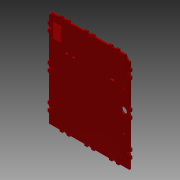
# Autodesk Inventor part: dolna_gt2_v2ipt
Saved by Autodesk Inventor 2013 (Build 170138000, 138)
## iProperties
Created: 2014-01-08
Part Number: dolna_gt2_v2ipt
Material: Generic
Document SubType Name: Modeling
Designer: dzban
Density: 1 g/cm^3
Author: dzban
Autodesk Inventor part; units mm, degrees
ref_plane "YZ Plane" through (0, 0, 0) normal (1, 0, 0) x (0, 1, 0)
ref_plane "XZ Plane" through (0, 0, 0) normal (0, 1, 0) x (-1, 0, 0)
ref_plane "XY Plane" through (0, 0, 0) normal (0, 0, 1) x (1, 0, 0)
sketch "Sketch1" plane through (0, 0, 0) normal (0, 1, 0) x (-1, 0, 0)
  line L0 (324.1317, 450.5892) -> (324.1317, 456.9892)
  line L1 (324.1317, 456.9892) -> (336.1317, 456.9892)
  line L2 (336.1317, 456.9892) -> (336.1317, 450.5892)
  line L3 (336.1317, 450.5892) -> (324.1317, 450.5892)
  line L4 (351.7317, 450.5892) -> (351.7317, 456.9892)
  line L5 (351.7317, 456.9892) -> (363.7317, 456.9892)
  line L6 (363.7317, 456.9892) -> (363.7317, 450.5892)
  line L7 (363.7317, 450.5892) -> (351.7317, 450.5892)
  arc A0 (416.5867, 566.9892) -> (427.5867, 555.9892) centre (427.5867, 566.9892) ccw
  line L8 (416.5867, 566.9892) -> (384.9367, 566.9892)
  line L9 (384.9367, 566.9892) -> (384.6367, 572.9892)
  line L10 (384.6367, 572.9892) -> (372.8367, 572.9892)
  line L11 (372.8367, 572.9892) -> (372.5367, 566.9892)
  line L12 (372.5367, 566.9892) -> (366.4367, 566.9892)
  line L13 (366.4367, 566.9892) -> (366.4367, 559.9892)
  line L14 (366.4367, 559.9892) -> (367.6867, 559.9892)
  line L15 (367.6867, 559.9892) -> (367.6867, 558.1892)
  line L16 (367.6867, 558.1892) -> (366.4367, 558.1892)
  line L17 (366.4367, 558.1892) -> (366.4367, 556.3892)
  line L18 (366.4367, 556.3892) -> (363.4367, 556.3892)
  line L19 (363.4367, 556.3892) -> (363.4367, 558.1892)
  line L20 (363.4367, 558.1892) -> (362.1867, 558.1892)
  line L21 (362.1867, 558.1892) -> (362.1867, 559.9892)
  line L22 (362.1867, 559.9892) -> (363.4367, 559.9892)
  line L23 (363.4367, 559.9892) -> (363.4367, 566.9892)
  line L24 (363.4367, 566.9892) -> (357.3367, 566.9892)
  line L25 (357.3367, 566.9892) -> (357.0367, 572.9892)
  line L26 (357.0367, 572.9892) -> (345.2367, 572.9892)
  line L27 (345.2367, 572.9892) -> (344.9367, 566.9892)
  line L28 (344.9367, 566.9892) -> (284.9367, 566.9892)
  line L29 (284.9367, 566.9892) -> (284.6367, 572.9892)
  line L30 (284.6367, 572.9892) -> (272.8367, 572.9892)
  line L31 (272.8367, 572.9892) -> (272.5367, 566.9892)
  line L32 (272.5367, 566.9892) -> (266.4367, 566.9892)
  line L33 (266.4367, 566.9892) -> (266.4367, 559.9892)
  line L34 (266.4367, 559.9892) -> (267.6867, 559.9892)
  line L35 (267.6867, 559.9892) -> (267.6867, 558.1892)
  line L36 (267.6867, 558.1892) -> (266.4367, 558.1892)
  line L37 (266.4367, 558.1892) -> (266.4367, 556.3892)
  line L38 (266.4367, 556.3892) -> (263.4367, 556.3892)
  line L39 (263.4367, 556.3892) -> (263.4367, 558.1892)
  line L40 (263.4367, 558.1892) -> (262.1867, 558.1892)
  line L41 (262.1867, 558.1892) -> (262.1867, 559.9892)
  line L42 (262.1867, 559.9892) -> (263.4367, 559.9892)
  line L43 (263.4367, 559.9892) -> (263.4367, 566.9892)
  line L44 (263.4367, 566.9892) -> (257.3367, 566.9892)
  line L45 (257.3367, 566.9892) -> (257.0367, 572.9892)
  line L46 (257.0367, 572.9892) -> (245.2367, 572.9892)
  line L47 (245.2367, 572.9892) -> (244.9367, 566.9892)
  line L48 (244.9367, 566.9892) -> (184.9367, 566.9892)
  line L49 (184.9367, 566.9892) -> (184.6367, 572.9892)
  line L50 (184.6367, 572.9892) -> (172.8367, 572.9892)
  line L51 (172.8367, 572.9892) -> (172.5367, 566.9892)
  line L52 (172.5367, 566.9892) -> (166.4367, 566.9892)
  line L53 (166.4367, 566.9892) -> (166.4367, 559.9892)
  line L54 (166.4367, 559.9892) -> (167.6867, 559.9892)
  line L55 (167.6867, 559.9892) -> (167.6867, 558.1892)
  line L56 (167.6867, 558.1892) -> (166.4367, 558.1892)
  line L57 (166.4367, 558.1892) -> (166.4367, 556.3892)
  line L58 (166.4367, 556.3892) -> (163.4367, 556.3892)
  line L59 (163.4367, 556.3892) -> (163.4367, 558.1892)
  line L60 (163.4367, 558.1892) -> (162.1867, 558.1892)
  line L61 (162.1867, 558.1892) -> (162.1867, 559.9892)
  line L62 (162.1867, 559.9892) -> (163.4367, 559.9892)
  line L63 (163.4367, 559.9892) -> (163.4367, 566.9892)
  line L64 (163.4367, 566.9892) -> (157.3367, 566.9892)
  line L65 (157.3367, 566.9892) -> (157.0367, 572.9892)
  line L66 (157.0367, 572.9892) -> (145.2367, 572.9892)
  line L67 (145.2367, 572.9892) -> (144.9367, 566.9892)
  line L68 (144.9367, 566.9892) -> (118.2867, 566.9892)
  arc A1 (102.2867, 550.9892) -> (118.2867, 566.9892) centre (102.2867, 566.9892) ccw
  line L69 (102.2867, 550.9892) -> (102.2867, 529.3892)
  line L70 (102.2867, 529.3892) -> (96.2867, 529.0892)
  line L71 (96.2867, 529.0892) -> (96.2867, 517.2892)
  line L72 (96.2867, 517.2892) -> (102.2867, 516.9892)
  line L73 (102.2867, 516.9892) -> (102.2867, 510.8892)
  line L74 (102.2867, 510.8892) -> (109.2867, 510.8892)
  line L75 (109.2867, 510.8892) -> (109.2867, 512.1392)
  line L76 (109.2867, 512.1392) -> (111.0867, 512.1392)
  line L77 (111.0867, 512.1392) -> (111.0867, 510.8892)
  line L78 (111.0867, 510.8892) -> (112.8867, 510.8892)
  line L79 (112.8867, 510.8892) -> (112.8867, 507.8892)
  line L80 (112.8867, 507.8892) -> (111.0867, 507.8892)
  line L81 (111.0867, 507.8892) -> (111.0867, 506.6392)
  line L82 (111.0867, 506.6392) -> (109.2867, 506.6392)
  line L83 (109.2867, 506.6392) -> (109.2867, 507.8892)
  line L84 (109.2867, 507.8892) -> (102.2867, 507.8892)
  line L85 (102.2867, 507.8892) -> (102.2867, 501.7892)
  line L86 (102.2867, 501.7892) -> (96.2867, 501.4892)
  line L87 (96.2867, 501.4892) -> (96.2867, 489.6892)
  line L88 (96.2867, 489.6892) -> (102.2867, 489.3892)
  line L89 (102.2867, 489.3892) -> (102.2867, 389.3892)
  line L90 (102.2867, 389.3892) -> (96.2867, 389.0892)
  line L91 (96.2867, 389.0892) -> (96.2867, 377.2892)
  line L92 (96.2867, 377.2892) -> (102.2867, 376.9892)
  line L93 (102.2867, 376.9892) -> (102.2867, 370.8892)
  line L94 (102.2867, 370.8892) -> (105.2867, 370.8892)
  line L95 (105.2867, 370.8892) -> (105.2867, 372.1392)
  line L96 (105.2867, 372.1392) -> (107.1867, 372.1392)
  line L97 (107.1867, 372.1392) -> (107.1867, 370.8892)
  line L98 (107.1867, 370.8892) -> (108.8867, 370.8892)
  line L99 (108.8867, 370.8892) -> (108.8867, 367.8892)
  line L100 (108.8867, 367.8892) -> (107.1867, 367.8892)
  line L101 (107.1867, 367.8892) -> (107.1867, 366.6392)
  line L102 (107.1867, 366.6392) -> (105.2867, 366.6392)
  line L103 (105.2867, 366.6392) -> (105.2867, 367.8892)
  line L104 (105.2867, 367.8892) -> (102.2867, 367.8892)
  line L105 (102.2867, 367.8892) -> (102.2867, 361.7892)
  line L106 (102.2867, 361.7892) -> (96.2867, 361.4892)
  line L107 (96.2867, 361.4892) -> (96.2867, 349.6892)
  line L108 (96.2867, 349.6892) -> (102.2867, 349.3892)
  line L109 (102.2867, 349.3892) -> (102.2867, 249.3892)
  line L110 (102.2867, 249.3892) -> (96.2867, 249.0892)
  line L111 (96.2867, 249.0892) -> (96.2867, 237.2892)
  line L112 (96.2867, 237.2892) -> (102.2867, 236.9892)
  line L113 (102.2867, 236.9892) -> (102.2867, 230.8892)
  line L114 (102.2867, 230.8892) -> (109.2867, 230.8892)
  line L115 (109.2867, 230.8892) -> (109.2867, 232.1392)
  line L116 (109.2867, 232.1392) -> (111.0867, 232.1392)
  line L117 (111.0867, 232.1392) -> (111.0867, 230.8892)
  line L118 (111.0867, 230.8892) -> (112.8867, 230.8892)
  line L119 (112.8867, 230.8892) -> (112.8867, 227.8892)
  line L120 (112.8867, 227.8892) -> (111.0867, 227.8892)
  line L121 (111.0867, 227.8892) -> (111.0867, 226.6392)
  line L122 (111.0867, 226.6392) -> (109.2867, 226.6392)
  line L123 (109.2867, 226.6392) -> (109.2867, 227.8892)
  line L124 (109.2867, 227.8892) -> (102.2867, 227.8892)
  line L125 (102.2867, 227.8892) -> (102.2867, 221.7892)
  line L126 (102.2867, 221.7892) -> (96.2867, 221.4892)
  line L127 (96.2867, 221.4892) -> (96.2867, 209.6892)
  line L128 (96.2867, 209.6892) -> (102.2867, 209.3892)
  line L129 (102.2867, 209.3892) -> (102.2867, 171.7892)
  line L130 (102.2867, 171.7892) -> (144.9367, 171.7892)
  line L131 (144.9367, 171.7892) -> (145.2367, 165.7892)
  line L132 (145.2367, 165.7892) -> (157.0367, 165.7892)
  line L133 (157.0367, 165.7892) -> (157.3367, 171.7892)
  line L134 (157.3367, 171.7892) -> (163.4367, 171.7892)
  line L135 (163.4367, 171.7892) -> (163.4367, 178.7892)
  line L136 (163.4367, 178.7892) -> (162.1867, 178.7892)
  line L137 (162.1867, 178.7892) -> (162.1867, 180.5892)
  line L138 (162.1867, 180.5892) -> (163.4367, 180.5892)
  line L139 (163.4367, 180.5892) -> (163.4367, 182.3892)
  line L140 (163.4367, 182.3892) -> (166.4367, 182.3892)
  line L141 (166.4367, 182.3892) -> (166.4367, 180.5892)
  line L142 (166.4367, 180.5892) -> (167.6867, 180.5892)
  line L143 (167.6867, 180.5892) -> (167.6867, 178.7892)
  line L144 (167.6867, 178.7892) -> (166.4367, 178.7892)
  line L145 (166.4367, 178.7892) -> (166.4367, 171.7892)
  line L146 (166.4367, 171.7892) -> (172.5367, 171.7892)
  line L147 (172.5367, 171.7892) -> (172.8367, 165.7892)
  line L148 (172.8367, 165.7892) -> (184.6367, 165.7892)
  line L149 (184.6367, 165.7892) -> (184.9367, 171.7892)
  line L150 (184.9367, 171.7892) -> (244.9367, 171.7892)
  line L151 (244.9367, 171.7892) -> (245.2367, 165.7892)
  line L152 (245.2367, 165.7892) -> (257.0367, 165.7892)
  line L153 (257.0367, 165.7892) -> (257.3367, 171.7892)
  line L154 (257.3367, 171.7892) -> (263.4367, 171.7892)
  line L155 (263.4367, 171.7892) -> (263.4367, 178.7892)
  line L156 (263.4367, 178.7892) -> (262.1867, 178.7892)
  line L157 (262.1867, 178.7892) -> (262.1867, 180.5892)
  line L158 (262.1867, 180.5892) -> (263.4367, 180.5892)
  line L159 (263.4367, 180.5892) -> (263.4367, 182.3892)
  line L160 (263.4367, 182.3892) -> (266.4367, 182.3892)
  line L161 (266.4367, 182.3892) -> (266.4367, 180.5892)
  line L162 (266.4367, 180.5892) -> (267.6867, 180.5892)
  line L163 (267.6867, 180.5892) -> (267.6867, 178.7892)
  line L164 (267.6867, 178.7892) -> (266.4367, 178.7892)
  line L165 (266.4367, 178.7892) -> (266.4367, 171.7892)
  line L166 (266.4367, 171.7892) -> (272.5367, 171.7892)
  line L167 (272.5367, 171.7892) -> (272.8367, 165.7892)
  line L168 (272.8367, 165.7892) -> (284.6367, 165.7892)
  line L169 (284.6367, 165.7892) -> (284.9367, 171.7892)
  line L170 (284.9367, 171.7892) -> (344.9367, 171.7892)
  line L171 (344.9367, 171.7892) -> (345.2367, 165.7892)
  line L172 (345.2367, 165.7892) -> (357.0367, 165.7892)
  line L173 (357.0367, 165.7892) -> (357.3367, 171.7892)
  line L174 (357.3367, 171.7892) -> (363.4367, 171.7892)
  line L175 (363.4367, 171.7892) -> (363.4367, 178.7892)
  line L176 (363.4367, 178.7892) -> (362.1867, 178.7892)
  line L177 (362.1867, 178.7892) -> (362.1867, 180.5892)
  line L178 (362.1867, 180.5892) -> (363.4367, 180.5892)
  line L179 (363.4367, 180.5892) -> (363.4367, 182.3892)
  line L180 (363.4367, 182.3892) -> (366.4367, 182.3892)
  line L181 (366.4367, 182.3892) -> (366.4367, 180.5892)
  line L182 (366.4367, 180.5892) -> (367.6867, 180.5892)
  line L183 (367.6867, 180.5892) -> (367.6867, 178.7892)
  line L184 (367.6867, 178.7892) -> (366.4367, 178.7892)
  line L185 (366.4367, 178.7892) -> (366.4367, 171.7892)
  line L186 (366.4367, 171.7892) -> (372.5367, 171.7892)
  line L187 (372.5367, 171.7892) -> (372.8367, 165.7892)
  line L188 (372.8367, 165.7892) -> (384.6367, 165.7892)
  line L189 (384.6367, 165.7892) -> (384.9367, 171.7892)
  line L190 (384.9367, 171.7892) -> (427.5867, 171.7892)
  line L191 (427.5867, 171.7892) -> (427.5867, 209.3892)
  line L192 (427.5867, 209.3892) -> (433.5867, 209.6892)
  line L193 (433.5867, 209.6892) -> (433.5867, 221.4892)
  line L194 (433.5867, 221.4892) -> (427.5867, 221.7892)
  line L195 (427.5867, 221.7892) -> (427.5867, 227.8892)
  line L196 (427.5867, 227.8892) -> (420.5867, 227.8892)
  line L197 (420.5867, 227.8892) -> (420.5867, 226.6392)
  line L198 (420.5867, 226.6392) -> (418.7867, 226.6392)
  line L199 (418.7867, 226.6392) -> (418.7867, 227.8892)
  line L200 (418.7867, 227.8892) -> (416.9867, 227.8892)
  line L201 (416.9867, 227.8892) -> (416.9867, 230.8892)
  line L202 (416.9867, 230.8892) -> (418.7867, 230.8892)
  line L203 (418.7867, 230.8892) -> (418.7867, 232.1392)
  line L204 (418.7867, 232.1392) -> (420.5867, 232.1392)
  line L205 (420.5867, 232.1392) -> (420.5867, 230.8892)
  line L206 (420.5867, 230.8892) -> (427.5867, 230.8892)
  line L207 (427.5867, 230.8892) -> (427.5867, 236.9892)
  line L208 (427.5867, 236.9892) -> (433.5867, 237.2892)
  line L209 (433.5867, 237.2892) -> (433.5867, 249.0892)
  line L210 (433.5867, 249.0892) -> (427.5867, 249.3892)
  line L211 (427.5867, 249.3892) -> (427.5867, 349.3892)
  line L212 (427.5867, 349.3892) -> (433.5867, 349.6892)
  line L213 (433.5867, 349.6892) -> (433.5867, 361.4892)
  line L214 (433.5867, 361.4892) -> (427.5867, 361.7892)
  line L215 (427.5867, 361.7892) -> (427.5867, 367.8892)
  line L216 (427.5867, 367.8892) -> (420.5867, 367.8892)
  line L217 (420.5867, 367.8892) -> (420.5867, 366.6392)
  line L218 (420.5867, 366.6392) -> (418.7867, 366.6392)
  line L219 (418.7867, 366.6392) -> (418.7867, 367.8892)
  line L220 (418.7867, 367.8892) -> (416.9867, 367.8892)
  line L221 (416.9867, 367.8892) -> (416.9867, 370.8892)
  line L222 (416.9867, 370.8892) -> (418.7867, 370.8892)
  line L223 (418.7867, 370.8892) -> (418.7867, 372.1392)
  line L224 (418.7867, 372.1392) -> (420.5867, 372.1392)
  line L225 (420.5867, 372.1392) -> (420.5867, 370.8892)
  line L226 (420.5867, 370.8892) -> (427.5867, 370.8892)
  line L227 (427.5867, 370.8892) -> (427.5867, 376.9892)
  line L228 (427.5867, 376.9892) -> (433.5867, 377.2892)
  line L229 (433.5867, 377.2892) -> (433.5867, 389.0892)
  line L230 (433.5867, 389.0892) -> (427.5867, 389.3892)
  line L231 (427.5867, 389.3892) -> (427.5867, 489.3892)
  line L232 (427.5867, 489.3892) -> (433.5867, 489.6892)
  line L233 (433.5867, 489.6892) -> (433.5867, 501.4892)
  line L234 (433.5867, 501.4892) -> (427.5867, 501.7892)
  line L235 (427.5867, 501.7892) -> (427.5867, 507.8892)
  line L236 (427.5867, 507.8892) -> (420.5867, 507.8892)
  line L237 (420.5867, 507.8892) -> (420.5867, 506.6392)
  line L238 (420.5867, 506.6392) -> (418.7867, 506.6392)
  line L239 (418.7867, 506.6392) -> (418.7867, 507.8892)
  line L240 (418.7867, 507.8892) -> (416.9867, 507.8892)
  line L241 (416.9867, 507.8892) -> (416.9867, 510.8892)
  line L242 (416.9867, 510.8892) -> (418.7867, 510.8892)
  line L243 (418.7867, 510.8892) -> (418.7867, 512.1392)
  line L244 (418.7867, 512.1392) -> (420.5867, 512.1392)
  line L245 (420.5867, 512.1392) -> (420.5867, 510.8892)
  line L246 (420.5867, 510.8892) -> (427.5867, 510.8892)
  line L247 (427.5867, 510.8892) -> (427.5867, 516.9892)
  line L248 (427.5867, 516.9892) -> (433.5867, 517.2892)
  line L249 (433.5867, 517.2892) -> (433.5867, 529.0892)
  line L250 (433.5867, 529.0892) -> (427.5867, 529.3892)
  line L251 (427.5867, 529.3892) -> (427.5867, 555.9892)
  arc A2 (379.1867, 487.3892) -> (380.5867, 485.9892) centre (380.5867, 487.3892) ccw
  line L252 (379.1867, 487.3892) -> (379.1867, 487.5892)
  arc A3 (380.5867, 488.9892) -> (379.1867, 487.5892) centre (380.5867, 487.5892) ccw
  line L253 (380.5867, 488.9892) -> (412.5867, 488.9892)
  arc A4 (413.9867, 487.5892) -> (412.5867, 488.9892) centre (412.5867, 487.5892) ccw
  line L254 (413.9867, 487.5892) -> (413.9867, 487.3892)
  arc A5 (412.5867, 485.9892) -> (413.9867, 487.3892) centre (412.5867, 487.3892) ccw
  line L255 (412.5867, 485.9892) -> (380.5867, 485.9892)
  arc A6 (413.9867, 499.5892) -> (412.5867, 500.9892) centre (412.5867, 499.5892) ccw
  line L256 (413.9867, 499.5892) -> (413.9867, 499.3892)
  arc A7 (412.5867, 497.9892) -> (413.9867, 499.3892) centre (412.5867, 499.3892) ccw
  line L257 (412.5867, 497.9892) -> (380.5867, 497.9892)
  arc A8 (379.1867, 499.3892) -> (380.5867, 497.9892) centre (380.5867, 499.3892) ccw
  line L258 (379.1867, 499.3892) -> (379.1867, 499.5892)
  arc A9 (380.5867, 500.9892) -> (379.1867, 499.5892) centre (380.5867, 499.5892) ccw
  line L259 (380.5867, 500.9892) -> (412.5867, 500.9892)
  arc A10 (413.9867, 511.5892) -> (412.5867, 512.9892) centre (412.5867, 511.5892) ccw
  line L260 (413.9867, 511.5892) -> (413.9867, 511.3892)
  arc A11 (412.5867, 509.9892) -> (413.9867, 511.3892) centre (412.5867, 511.3892) ccw
  line L261 (412.5867, 509.9892) -> (380.5867, 509.9892)
  arc A12 (379.1867, 511.3892) -> (380.5867, 509.9892) centre (380.5867, 511.3892) ccw
  line L262 (379.1867, 511.3892) -> (379.1867, 511.5892)
  arc A13 (380.5867, 512.9892) -> (379.1867, 511.5892) centre (380.5867, 511.5892) ccw
  line L263 (380.5867, 512.9892) -> (412.5867, 512.9892)
  arc A14 (413.9867, 523.5892) -> (412.5867, 524.9892) centre (412.5867, 523.5892) ccw
  line L264 (413.9867, 523.5892) -> (413.9867, 523.3892)
  arc A15 (412.5867, 521.9892) -> (413.9867, 523.3892) centre (412.5867, 523.3892) ccw
  line L265 (412.5867, 521.9892) -> (380.5867, 521.9892)
  arc A16 (379.1867, 523.3892) -> (380.5867, 521.9892) centre (380.5867, 523.3892) ccw
  line L266 (379.1867, 523.3892) -> (379.1867, 523.5892)
  arc A17 (380.5867, 524.9892) -> (379.1867, 523.5892) centre (380.5867, 523.5892) ccw
  line L267 (380.5867, 524.9892) -> (412.5867, 524.9892)
  arc A18 (413.9867, 535.5892) -> (412.5867, 536.9892) centre (412.5867, 535.5892) ccw
  line L268 (413.9867, 535.5892) -> (413.9867, 535.3892)
  arc A19 (412.5867, 533.9892) -> (413.9867, 535.3892) centre (412.5867, 535.3892) ccw
  line L269 (412.5867, 533.9892) -> (380.5867, 533.9892)
  arc A20 (379.1867, 535.3892) -> (380.5867, 533.9892) centre (380.5867, 535.3892) ccw
  line L270 (379.1867, 535.3892) -> (379.1867, 535.5892)
  arc A21 (380.5867, 536.9892) -> (379.1867, 535.5892) centre (380.5867, 535.5892) ccw
  line L271 (380.5867, 536.9892) -> (412.5867, 536.9892)
  line L272 (182.0547, 456.9892) -> (182.0547, 450.5892)
  line L273 (182.0547, 450.5892) -> (164.4547, 450.5892)
  line L274 (164.4547, 450.5892) -> (164.4547, 456.9892)
  line L275 (164.4547, 456.9892) -> (182.0547, 456.9892)
  arc A22 (413.9867, 529.5892) -> (412.5867, 530.9892) centre (412.5867, 529.5892) ccw
  line L276 (413.9867, 529.5892) -> (413.9867, 529.3892)
  arc A23 (412.5867, 527.9892) -> (413.9867, 529.3892) centre (412.5867, 529.3892) ccw
  line L277 (412.5867, 527.9892) -> (380.5867, 527.9892)
  arc A24 (379.1867, 529.3892) -> (380.5867, 527.9892) centre (380.5867, 529.3892) ccw
  line L278 (379.1867, 529.3892) -> (379.1867, 529.5892)
  arc A25 (380.5867, 530.9892) -> (379.1867, 529.5892) centre (380.5867, 529.5892) ccw
  line L279 (380.5867, 530.9892) -> (412.5867, 530.9892)
  arc A26 (413.9867, 517.5892) -> (412.5867, 518.9892) centre (412.5867, 517.5892) ccw
  line L280 (413.9867, 517.5892) -> (413.9867, 517.3892)
  arc A27 (412.5867, 515.9892) -> (413.9867, 517.3892) centre (412.5867, 517.3892) ccw
  line L281 (412.5867, 515.9892) -> (380.5867, 515.9892)
  arc A28 (379.1867, 517.3892) -> (380.5867, 515.9892) centre (380.5867, 517.3892) ccw
  line L282 (379.1867, 517.3892) -> (379.1867, 517.5892)
  arc A29 (380.5867, 518.9892) -> (379.1867, 517.5892) centre (380.5867, 517.5892) ccw
  line L283 (380.5867, 518.9892) -> (412.5867, 518.9892)
  arc A30 (413.9867, 505.5892) -> (412.5867, 506.9892) centre (412.5867, 505.5892) ccw
  line L284 (413.9867, 505.5892) -> (413.9867, 505.3892)
  arc A31 (412.5867, 503.9892) -> (413.9867, 505.3892) centre (412.5867, 505.3892) ccw
  line L285 (412.5867, 503.9892) -> (380.5867, 503.9892)
  arc A32 (379.1867, 505.3892) -> (380.5867, 503.9892) centre (380.5867, 505.3892) ccw
  line L286 (379.1867, 505.3892) -> (379.1867, 505.5892)
  arc A33 (380.5867, 506.9892) -> (379.1867, 505.5892) centre (380.5867, 505.5892) ccw
  line L287 (380.5867, 506.9892) -> (412.5867, 506.9892)
  arc A34 (413.9867, 493.5892) -> (412.5867, 494.9892) centre (412.5867, 493.5892) ccw
  line L288 (413.9867, 493.5892) -> (413.9867, 493.3892)
  arc A35 (412.5867, 491.9892) -> (413.9867, 493.3892) centre (412.5867, 493.3892) ccw
  line L289 (412.5867, 491.9892) -> (380.5867, 491.9892)
  arc A36 (379.1867, 493.3892) -> (380.5867, 491.9892) centre (380.5867, 493.3892) ccw
  line L290 (379.1867, 493.3892) -> (379.1867, 493.5892)
  arc A37 (380.5867, 494.9892) -> (379.1867, 493.5892) centre (380.5867, 493.5892) ccw
  line L291 (380.5867, 494.9892) -> (412.5867, 494.9892)
  arc A38 (413.9867, 481.5892) -> (412.5867, 482.9892) centre (412.5867, 481.5892) ccw
  line L292 (413.9867, 481.5892) -> (413.9867, 481.3892)
  arc A39 (412.5867, 479.9892) -> (413.9867, 481.3892) centre (412.5867, 481.3892) ccw
  line L293 (412.5867, 479.9892) -> (380.5867, 479.9892)
  arc A40 (379.1867, 481.3892) -> (380.5867, 479.9892) centre (380.5867, 481.3892) ccw
  line L294 (379.1867, 481.3892) -> (379.1867, 481.5892)
  arc A41 (380.5867, 482.9892) -> (379.1867, 481.5892) centre (380.5867, 481.5892) ccw
  line L295 (380.5867, 482.9892) -> (412.5867, 482.9892)
  arc A42 (121.2867, 380.3892) -> (121.2867, 358.3892) centre (121.2867, 369.3892) ccw
  line L296 (121.2867, 380.3892) -> (127.2867, 380.3892)
  arc A43 (127.2867, 358.3892) -> (127.2867, 380.3892) centre (127.2867, 369.3892) ccw
  line L297 (127.2867, 358.3892) -> (121.2867, 358.3892)
  line L298 (112.7867, 352.3892) -> (106.7867, 352.3892)
  arc A44 (106.7867, 355.3892) -> (106.7867, 352.3892) centre (106.7867, 353.8892) ccw
  line L299 (106.7867, 355.3892) -> (112.7867, 355.3892)
  arc A45 (112.7867, 352.3892) -> (112.7867, 355.3892) centre (112.7867, 353.8892) ccw
  line L300 (143.7867, 352.3892) -> (137.7867, 352.3892)
  arc A46 (137.7867, 355.3892) -> (137.7867, 352.3892) centre (137.7867, 353.8892) ccw
  line L301 (137.7867, 355.3892) -> (143.7867, 355.3892)
  arc A47 (143.7867, 352.3892) -> (143.7867, 355.3892) centre (143.7867, 353.8892) ccw
  line L302 (112.7867, 383.3892) -> (106.7867, 383.3892)
  arc A48 (106.7867, 386.3892) -> (106.7867, 383.3892) centre (106.7867, 384.8892) ccw
  line L303 (106.7867, 386.3892) -> (112.7867, 386.3892)
  arc A49 (112.7867, 383.3892) -> (112.7867, 386.3892) centre (112.7867, 384.8892) ccw
  line L304 (143.7867, 383.3892) -> (137.7867, 383.3892)
  arc A50 (137.7867, 386.3892) -> (137.7867, 383.3892) centre (137.7867, 384.8892) ccw
  line L305 (137.7867, 386.3892) -> (143.7867, 386.3892)
  arc A51 (143.7867, 383.3892) -> (143.7867, 386.3892) centre (143.7867, 384.8892) ccw
  circle A52 centre (124.2867, 300.3892) radius 1.5
  circle A53 centre (124.2867, 460.3892) radius 1.5
  circle A54 centre (124.2867, 438.3892) radius 1.5
  circle A55 centre (124.2867, 278.3892) radius 1.5
  circle A56 centre (124.2867, 289.3892) radius 3.95
  circle A57 centre (124.2867, 449.3892) radius 3.95
  circle A58 centre (382.5867, 554.7892) radius 1.5
  circle A59 centre (203.2867, 493.1892) radius 1.5
  circle A60 centre (142.2867, 559.9892) radius 1.5
  circle A61 centre (176.0867, 370.8392) radius 1.5
  circle A62 centre (356.1317, 497.5772) radius 1.5
  circle A63 centre (271.0417, 497.5772) radius 1.5
  circle A64 centre (245.9367, 453.7892) radius 1.5
  circle A65 centre (176.0867, 364.8392) radius 1.5
  circle A66 centre (142.2867, 553.9892) radius 1.5
  circle A67 centre (197.2867, 493.1892) radius 1.5
  circle A68 centre (382.5867, 548.7892) radius 1.5
  circle A69 centre (343.9317, 453.7892) radius 1.5
  circle A70 centre (356.1317, 555.4892) radius 1.5
  circle A71 centre (282.7257, 555.4892) radius 1.5
  point P0 (0, 0)
  dimension "d0" = 171.7892
  dimension "d1" = 102.2867
  dimension "d2" = 395.2
  dimension "d6" = 6
  dimension "d54" = 6
  dimension "d55" = 6
  dimension "d56" = 16
  dimension "d57" = 11
  dimension "d58" = 7
  dimension "d59" = 1.8
  dimension "d60" = 1.8
  dimension "d62" = 11.8
  dimension "d63" = 12.4
  dimension "d64" = 0.3
  dimension "d65" = 6.1
  dimension "d66" = 6.1
  dimension "d67" = 3
  dimension "d68" = 1.25
  dimension "d69" = 1.25
  dimension "d70" = 12.4
  dimension "d71" = 100
  dimension "d72" = 6.1
  dimension "d73" = 12.4
  dimension "d74" = 3
  dimension "d75" = 1.25
  dimension "d76" = 1.25
  dimension "d77" = 100
  dimension "d78" = 6.1
  dimension "d79" = 12.4
  dimension "d80" = 6.1
  dimension "d81" = 12.4
  dimension "d82" = 3
  dimension "d83" = 1.25
  dimension "d84" = 1.25
  dimension "d85" = 6.1
  dimension "d86" = 11.8
  dimension "d87" = 10.6
  dimension "d88" = 1.8
  dimension "d89" = 1.8
  dimension "d90" = 6
  dimension "d92" = 12.4
  dimension "d93" = 6.1
  dimension "d94" = 3
  dimension "d95" = 6.1
  dimension "d96" = 12.4
  dimension "d97" = 1.25
  dimension "d98" = 1.25
  dimension "d99" = 10.6
  dimension "d100" = 7
  dimension "d101" = 1.8
  dimension "d102" = 140
  dimension "d103" = 6.1
  dimension "d104" = 12.4
  dimension "d105" = 6.1
  dimension "d106" = 12.4
  dimension "d107" = 3
  dimension "d108" = 1.25
  dimension "d109" = 1.25
  dimension "d110" = 140
  dimension "d111" = 6.1
  dimension "d112" = 12.4
  dimension "d113" = 6.1
  dimension "d114" = 3
  dimension "d115" = 12.4
  constraints: 612 end point, 210 parallel, 153 collinear, 136 tangent, 104 point on circle, 74 perpendicular, 72 centre point, 65 equal radius, 64 vertical alignment, 25 horizontal alignment, 1 horizontal
  measures "d0" distance from line of L130 point (0, 0)
  measures "d1" distance from line of point (0, 0) L129
  measures "d2" distance between parallel lines of L68 L130
  measures "d6" distance between parallel lines of L109 L111
  measures "d54" distance between parallel lines of L130 L132
  measures "d55" distance between parallel lines of L66 L68
  measures "d56" radius of A1
  measures "d57" radius of A0
  measures "d58" distance between parallel lines of L136 L134
  measures "d59" distance between parallel lines of L138 L136
  measures "d60" distance between parallel lines of L140 L138
  measures "d62" distance of L131.end L132.end
  measures "d63" distance of L133.end L130.end
  measures "d64" horizontal distance of L130.end L131.end
  measures "d65" distance of L134.end L133.end
  measures "d66" distance of L146.end L145.end
  measures "d67" distance between parallel lines of L145 L135
  measures "d68" distance between parallel lines of L137 L135
  measures "d69" distance between parallel lines of L143 L145
  measures "d70" distance of L149.end L146.end
  measures "d71" distance between parallel lines of L155 L135
  measures "d72" distance of L154.end L153.end
  measures "d73" distance of L150.end L153.end
  measures "d74" distance between parallel lines of L165 L155
  measures "d75" distance between parallel lines of L163 L165
  measures "d76" distance between parallel lines of L157 L155
  measures "d77" distance between parallel lines of L175 L155
  measures "d78" distance of L165.end L166.end
  measures "d79" distance of L169.end L166.end
  measures "d80" distance of L173.end L174.end
  measures "d81" distance of L170.end L173.end
  measures "d82" distance between parallel lines of L185 L175
  measures "d83" distance between parallel lines of L177 L175
  measures "d84" distance between parallel lines of L183 L185
  measures "d85" distance of L185.end L186.end
  measures "d86" distance of L187.end L188.end
  measures "d87" distance between parallel lines of L64 L58
  measures "d88" distance from line of L60.end L58
  measures "d89" distance between parallel lines of L62 L60
  measures "d90" distance between parallel lines of L233 L231
  measures "d92" distance of L250.end L247.end
  measures "d93" distance from line of L247.end L246
  measures "d94" distance between parallel lines of L246 L236
  measures "d95" distance from line of L236 L234.end
  measures "d96" distance of L234.end L231.end
  measures "d97" distance between parallel lines of L240 L238
  measures "d98" distance between parallel lines of L244 L242
  measures "d99" distance between parallel lines of L247 L241
  measures "d100" distance between parallel lines of L247 L245
  measures "d101" distance between parallel lines of L245 L243
  measures "d102" distance between parallel lines of L226 L246
  measures "d103" distance of L226.end L227.end
  measures "d104" distance of L230.end L227.end
  measures "d105" distance of L214.end L215.end
  measures "d106" distance of L214.end L211.end
  measures "d107" distance between parallel lines of L226 L216
  measures "d108" distance between parallel lines of L224 L222
  measures "d109" distance between parallel lines of L220 L218
  measures "d110" distance between parallel lines of L206 L226
  measures "d111" distance of L206.end L207.end
  measures "d112" distance of L210.end L207.end
  measures "d113" distance of L194.end L195.end
  measures "d114" distance between parallel lines of L206 L196
  measures "d115" distance of L194.end L191.end
extrude "Extrusion1" add sketch "Sketch1" along normal blind 6
sketch "Sketch2" plane through (0, 0, 0) normal (0, -1, 0) x (1, 0, 0)
  line L0 (-127.2867, 380.3892) -> (-121.2867, 380.3892) projected
  arc A0 (-121.2867, 358.3892) -> (-121.2867, 380.3892) centre (-121.2867, 369.3892) ccw projected
  line L1 (-121.2867, 358.3892) -> (-127.2867, 358.3892) projected
  arc A1 (-127.2867, 380.3892) -> (-127.2867, 358.3892) centre (-127.2867, 369.3892) ccw projected
  arc A2 (-137.7867, 383.3892) -> (-137.7867, 386.3892) centre (-137.7867, 384.8892) ccw projected
  line L2 (-137.7867, 383.3892) -> (-143.7867, 383.3892) projected
  arc A3 (-143.7867, 386.3892) -> (-143.7867, 383.3892) centre (-143.7867, 384.8892) ccw projected
  line L3 (-143.7867, 386.3892) -> (-137.7867, 386.3892) projected
  arc A4 (-106.7867, 383.3892) -> (-106.7867, 386.3892) centre (-106.7867, 384.8892) ccw projected
  line L4 (-106.7867, 383.3892) -> (-112.7867, 383.3892) projected
  arc A5 (-112.7867, 386.3892) -> (-112.7867, 383.3892) centre (-112.7867, 384.8892) ccw projected
  line L5 (-112.7867, 386.3892) -> (-106.7867, 386.3892) projected
  arc A6 (-137.7867, 352.3892) -> (-137.7867, 355.3892) centre (-137.7867, 353.8892) ccw projected
  line L6 (-137.7867, 352.3892) -> (-143.7867, 352.3892) projected
  arc A7 (-143.7867, 355.3892) -> (-143.7867, 352.3892) centre (-143.7867, 353.8892) ccw projected
  line L7 (-143.7867, 355.3892) -> (-137.7867, 355.3892) projected
  arc A8 (-106.7867, 352.3892) -> (-106.7867, 355.3892) centre (-106.7867, 353.8892) ccw projected
  line L8 (-106.7867, 352.3892) -> (-112.7867, 352.3892) projected
  arc A9 (-112.7867, 355.3892) -> (-112.7867, 352.3892) centre (-112.7867, 353.8892) ccw projected
  line L9 (-112.7867, 355.3892) -> (-106.7867, 355.3892) projected
  circle A10 centre (-140.7867, 384.8892) radius 1.5
  circle A11 centre (-109.7867, 384.8892) radius 1.5
  circle A12 centre (-109.7867, 353.8892) radius 1.5
  circle A13 centre (-140.7867, 353.8892) radius 1.5
  circle A14 centre (-124.2867, 369.3892) radius 11
  point P0 (0, 0)
  dimension "d144" = 3
  dimension "d146" = 3
  dimension "d147" = 3
  dimension "d148" = 22
  dimension "d149" = 3
  dimension "d150" = 3
  constraints: 5 centre point, 5 horizontal alignment, 2 tangent, 2 vertical alignment
  measures "d144" diameter of A12
  measures "d146" distance of A10.centre A2.centre
  measures "d147" distance of A11.centre A5.centre
  measures "d148" diameter of A14
  measures "d149" distance of A1.centre A14.centre
  measures "d150" diameter of A11
extrude "Extrusion2" add sketch "Sketch2" against normal blind 6 contours L0 A14 L1 A1 | L0 A0 L1 A14 | L2 A10 L3 A2 | L2 A3 L3 A10 | L4 A11 L5 A4 | L4 A5 L5 A11 | L6 A13 L7 A6 | L6 A7 L7 A13 | L8 A12 L9 A8 | L8 A9 L9 A12
sketch "Sketch3" plane through (0, 0, 0) normal (0, -1, 0) x (1, 0, 0)
  circle A0 centre (-124.2867, 369.3892) radius 11 projected
  circle A1 centre (-124.2867, 369.3892) radius 12
  point P0 (0, 0)
  dimension "d207" = 24
  constraints: 1 centre point, 1 coincident
  measures "d207" diameter of A1
extrude "Extrusion3" cut sketch "Sketch3" against normal blind 10
body "Solid1"
